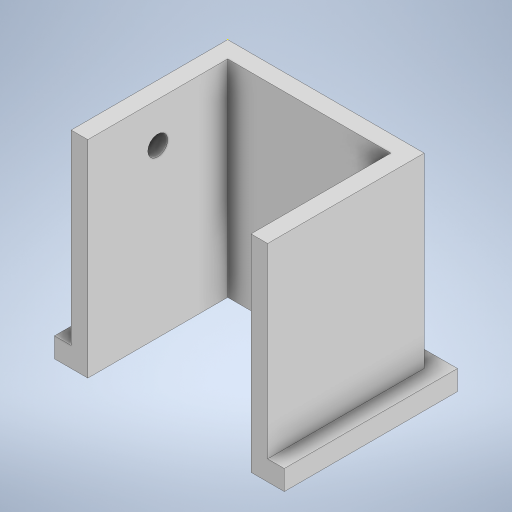
# Autodesk Inventor part: top cam mount v03
Saved by Autodesk Inventor 2023 (Build 270158000, 158)
## iProperties
Created: 2024-07-05
Part Number: top cam mount v03
Material: Generic
Document SubType Name: Modeling
Designer: Akramilab
Density: 1 g/cm^3
Appearance: Default
Author: Akramilab
Autodesk Inventor part; units mm, degrees
ref_plane "YZ Plane" through (0, 0, 0) normal (1, 0, 0) x (0, 1, 0)
ref_plane "XZ Plane" through (0, 0, 0) normal (0, 1, 0) x (-1, 0, 0)
ref_plane "XY Plane" through (0, 0, 0) normal (0, 0, 1) x (1, 0, 0)
sketch "Sketch1" plane through (0, 0, 0) normal (0, 1, 0) x (-1, 0, 0)
  line L0 (0, 0) -> (-59, 0)
  line L1 (-59, 0) -> (-59, 5)
  line L2 (-59, 5) -> (0, 5)
  line L3 (0, 5) -> (0, 0)
  line L4 (0, 5) -> (-5, 5)
  line L5 (-5, 5) -> (-5, 47)
  line L6 (-5, 47) -> (0, 47)
  line L7 (0, 47) -> (0, 5)
  line L8 (-59, 5) -> (-54, 5)
  line L9 (-54, 5) -> (-54, 47)
  line L10 (-54, 47) -> (-59, 47)
  line L11 (-59, 47) -> (-59, 5)
  point P0 (-54, 5)
  dimension "d0" = 59
  dimension "d1" = 5
  dimension "d2" = 5
  dimension "d3" = 42
  dimension "d4" = 5
  dimension "d5" = 42
  constraints: 24 end point, 6 parallel, 3 horizontal, 3 perpendicular
  measures "d0" distance of L1.end L2.end
  measures "d1" distance of L0.end L1.end
  measures "d2" distance of L5.end L6.end
  measures "d3" distance of L4.end L5.end
  measures "d4" distance of L10.end L9.end
  measures "d5" distance of L9.end L8.end
extrude "Extrusion1" add sketch "Sketch1" against normal blind 62
sketch "Sketch7" plane through (0, -62, 0) normal (0, -1, 0) x (1, 0, 0)
  line L0 (0, 47) -> (0, 0) projected
  line L1 (0, 47) -> (-5, 47)
  line L2 (-5, 47) -> (-5, -5)
  line L3 (-5, -5) -> (0, -5)
  line L4 (0, -5) -> (0, 47)
  line L5 (59, 47) -> (54, 47) projected
  line L6 (59, 47) -> (64, 47)
  line L7 (64, 47) -> (64, -5)
  line L8 (64, -5) -> (59, -5)
  line L9 (59, -5) -> (59, 47)
  line L10 (0, 0) -> (59, 0) projected
  line L11 (59, -5) -> (0, -5)
  line L12 (0, -5) -> (0, 0)
  line L13 (0, 0) -> (59, 0)
  line L14 (59, 0) -> (59, -5)
  dimension "d34" = 5
  dimension "d35" = 52
  dimension "d36" = 5
  dimension "d37" = 52
  constraints: 24 end point, 6 parallel, 3 horizontal, 3 perpendicular
  measures "d34" distance of L3.end L2.end
  measures "d35" distance of L2.end L1.end
  measures "d36" distance of L7.end L8.end
  measures "d37" distance of L6.end L7.end
extrude "Extrusion7" add sketch "Sketch7" against normal blind 6
sketch "Sketch8" plane through (0, -62, 0) normal (0, -1, 0) x (1, 0, 0)
  line L0 (0, 0) -> (0, 47) projected
  line L1 (5, 47) -> (-5, 47) projected
  circle A0 centre (0, 37) radius 2.5
  line L2 (59, 47) -> (59, 0) projected
  line L3 (64, 47) -> (54, 47) projected
  circle A1 centre (59, 37) radius 2.5
  line L4 (59, 0) -> (0, 0) projected
  line L5 (-5, 47) -> (-5, -5) projected
  line L6 (64, -5) -> (64, 47) projected
  circle A2 centre (16, 0) radius 2.5
  circle A3 centre (43, 0) radius 2.5
  point P0 (29.5, 0)
  dimension "d40" = 10
  dimension "d41" = 5
  dimension "d42" = 10
  dimension "d43" = 5
  dimension "d44" = 34.5
  dimension "d45" = 21
  dimension "d46" = 21
  dimension "d47" = 5
  dimension "d48" = 5
  constraints: 4 centre point, 4 coincident, 4 point on line, 1 midpoint
  measures "d40" distance from line of point (0, 37) L1
  measures "d41" diameter of A0
  measures "d42" distance from line of point (59, 37) L3
  measures "d43" diameter of A1
  measures "d44" distance from line of L5 point (29.5, 0)
  measures "d45" distance from line of point (16, 0) L5
  measures "d46" distance from line of point (43, 0) L6
  measures "d47" diameter of A2
  measures "d48" diameter of A3
extrude "Extrusion8" cut sketch "Sketch8" against normal blind 5
sketch "Sketch9" plane through (0, 0, 0) normal (-1, 0, 0) x (0, 0, 1)
  point P0 (0, 0)
sketch "Sketch10" plane through (0, 0, 0) normal (-1, 0, 0) x (0, 0, 1)
  line L0 (47, 0) -> (47, -56) projected
  line L1 (47, -62) -> (-5, -62) projected
  circle A0 centre (26, -12) radius 3
  point P0 (0, 0)
  dimension "d51" = 21
  dimension "d52" = 50
  dimension "d53" = 6
  constraints: 1 centre point, 1 coincident
  measures "d51" distance from line of L0 point (26, -12)
  measures "d52" distance from line of L1 point (26, -12)
  measures "d53" diameter of A0
extrude "Extrusion9" cut sketch "Sketch10" against normal blind 5
equation "\"d4\" = d2"
equation "\"d5\" = d3"
equation "\"d42\" = d40"
equation "\"d43\" = d41"
equation "\"d46\" = d45"
equation "\"d47\" = d41"
equation "\"d48\" = d47"
body "Solid1"
